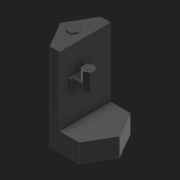
# Autodesk Inventor part: body
Saved by Autodesk Inventor 2017 (Build 210142000, 142)
## iProperties
Created: 2019-08-03
Part Number: body
Material: ABS Plastic
Document SubType Name: Modeling
Designer: Dell
Density: 1.06 g/cm^3
Appearance: Smooth - Black
Author: Dell
Autodesk Inventor part; units mm, degrees
ref_plane "YZ Plane" through (0, 0, 0) normal (1, 0, 0) x (0, 1, 0)
ref_plane "XZ Plane" through (0, 0, 0) normal (0, 1, 0) x (-1, 0, 0)
ref_plane "XY Plane" through (0, 0, 0) normal (0, 0, 1) x (1, 0, 0)
sketch "Sketch1" plane through (0, 0, 0) normal (0, 0, 1) x (1, 0, 0)
  line L0 (303.011, 0) -> (151.5055, -262.4152)
  line L1 (151.5055, -262.4152) -> (-151.5055, -262.4152)
  line L2 (-151.5055, -262.4152) -> (-303.011, 0)
  line L3 (-303.011, 0) -> (-151.5055, 262.4152)
  line L4 (-151.5055, 262.4152) -> (151.5055, 262.4152)
  line L5 (151.5055, 262.4152) -> (303.011, 0)
  point P0 (0, 0)
  point P1 (0, 0)
  dimension "d0" = 606.022
  constraints: 12 end point, 1 coincident, 1 horizontal alignment, 13 other
  measures "d0" distance of L2.end L0.start
extrude "Extrusion1" add sketch "Sketch1" along normal blind 190.5
sketch "Sketch2" plane through (0, 0, 190.5) normal (0, 0, 1) x (1, 0, 0)
  line L0 (151.5055, -262.4152) -> (303.011, 0) projected
  line L1 (303.011, 0) -> (151.5055, 262.4152) projected
  line L2 (151.5055, 262.4152) -> (-151.5055, 262.4152) construction
  line L3 (-151.5055, 262.4152) -> (-303.011, 0) projected
  line L4 (-303.011, 0) -> (-151.5055, -262.4152) projected
  line L5 (-151.5055, -262.4152) -> (151.5055, -262.4152) construction
  line L6 (151.5055, 262.4152) -> (-151.5055, 262.4152) projected
  line L7 (-50.7278, 262.4152) -> (-50.7278, -262.4152)
  line L8 (-151.5055, -262.4152) -> (151.5055, -262.4152) projected
  line L9 (-50.7278, 262.4152) -> (-151.5055, 262.4152)
  line L10 (-50.7278, -262.4152) -> (-151.5055, -262.4152)
  point P0 (0, 0)
  dimension "d3" = 353.7388
  constraints: 6 end point, 2 collinear, 2 point on line, 1 perpendicular
  measures "d3" distance from line of L0.end L7
extrude "Extrusion2" add sketch "Sketch2" along normal blind 704.85 contours L8 L4 L3 L6 L7
sketch "Sketch3" plane through (-50.7278, -262.4152, 190.5) normal (1, 0, 0) x (0, 0, -1)
  line L0 (-428.7, 86.64) -> (-358.7, 86.64)
  line L1 (-358.7, 86.64) -> (-358.7, 251.64)
  line L2 (-358.7, 251.64) -> (-428.7, 251.64)
  line L3 (-428.7, 251.64) -> (-428.7, 86.64)
  line L4 (0, 0) -> (-704.85, 0) projected
  line L5 (0, 0) -> (0, 262.4152) projected
  point P0 (190.5, 262.4152)
  dimension "d6" = 86.64
  dimension "d7" = 358.7
  dimension "d8" = 70
  dimension "d9" = 165
  constraints: 8 end point, 2 parallel, 1 horizontal, 1 perpendicular
  measures "d6" distance between parallel lines of L0 L4
  measures "d7" distance between parallel lines of L5 L1
  measures "d8" distance of L0.start L0.end
  measures "d9" distance of L2.end L0.start
extrude "Extrusion3" add sketch "Sketch3" along normal blind 30
sketch "Sketch4" plane through (-20.7278, -262.4152, 190.5) normal (1, 0, 0) x (0, 0, -1)
  line L0 (-428.7, 86.64) -> (-428.7, 251.64) projected
  line L1 (-358.7, 251.64) -> (-358.7, 86.64) projected
  line L2 (-428.7, 111.64) -> (-358.7, 111.64)
  line L3 (-358.7, 111.64) -> (-358.7, 226.64)
  line L4 (-358.7, 226.64) -> (-428.7, 226.64)
  line L5 (-428.7, 226.64) -> (-428.7, 111.64)
  point P0 (190.5, 262.4152)
  point P1 (-428.7, 169.14)
  dimension "d12" = 115
  constraints: 8 end point, 2 midpoint, 2 parallel, 2 point on line, 1 horizontal, 1 perpendicular
  measures "d12" distance between parallel lines of L4 L2
extrude "Extrusion4" add sketch "Sketch4" along normal blind 98.2
sketch "Sketch5" plane through (-50.7278, -175.7752, 619.2) normal (0, 0, 1) x (1, 0, 0)
  line L0 (128.2, 25) -> (128.2, 140) projected
  line L1 (128.2, 140) -> (177.9965, 111.25)
  line L2 (177.9965, 111.25) -> (177.9965, 53.75)
  line L3 (177.9965, 53.75) -> (128.2, 25)
  line L4 (128.2, 25) -> (78.4035, 53.75)
  line L5 (78.4035, 53.75) -> (78.4035, 111.25)
  line L6 (78.4035, 111.25) -> (128.2, 140)
  point P0 (50.7278, 175.7752)
  point P1 (128.2, 82.5)
  constraints: 12 end point, 1 midpoint, 13 other
extrude "Extrusion5" add sketch "Sketch5" along normal blind 110 and the other way blind 70
sketch "Sketch6" plane through (0, 0, 895.35) normal (0, 0, 1) x (1, 0, 0)
  line L0 (-115.8774, 0) -> (-144.6274, -49.7965)
  line L1 (-144.6274, -49.7965) -> (-202.1274, -49.7965)
  line L2 (-202.1274, -49.7965) -> (-230.8774, 0)
  line L3 (-230.8774, 0) -> (-202.1274, 49.7965)
  line L4 (-202.1274, 49.7965) -> (-144.6274, 49.7965)
  line L5 (-144.6274, 49.7965) -> (-115.8774, 0)
  line L6 (-50.7278, -262.4152) -> (-50.7278, 262.4152) projected
  point P0 (0, 0)
  point P1 (-173.3774, 0)
  point P2 (-50.7278, 0)
  dimension "d19" = 115
  dimension "d20" = 122.6496
  constraints: 12 end point, 2 horizontal alignment, 1 midpoint, 13 other
  measures "d19" distance of L0.start L2.end
  measures "d20" distance from line of L6 point (-173.377, 0)
extrude "Extrusion6" add sketch "Sketch6" along normal blind 11.725
sketch "Sketch7" plane through (-50.7278, -175.7752, 729.2) normal (0, 0, 1) x (1, 0, 0)
  line L0 (177.9965, 111.25) -> (128.2, 140) projected
  line L1 (128.2, 140) -> (78.4035, 111.25) projected
  line L2 (78.4035, 111.25) -> (78.4035, 53.75) projected
  line L3 (78.4035, 53.75) -> (128.2, 25) projected
  line L4 (128.2, 25) -> (177.9965, 53.75) projected
  line L5 (177.9965, 53.75) -> (177.9965, 111.25) projected
  circle A0 centre (128.2, 82.5) radius 25
  point P0 (50.7278, 175.7752)
  point P1 (177.9965, 82.5)
  dimension "d23" = 50
  constraints: 1 centre point, 1 horizontal alignment, 1 midpoint, 1 vertical alignment
  measures "d23" diameter of A0
extrude "Extrusion7" add sketch "Sketch7" along normal blind 5 contours A0
sketch "Sketch8" plane through (-151.5055, -262.4152, 0) normal (0, -1, 0) x (1, 0, 0)
  line L0 (303.011, 0) -> (0, 0) projected
  line L1 (303.011, 0) -> (303.011, 190.5) projected
  line L2 (100.7777, 190.5) -> (303.011, 190.5) projected
  line L3 (100.7777, 190.5) -> (100.7777, 895.35) projected
  line L4 (0, 895.35) -> (100.7777, 895.35) projected
  line L5 (0, 0) -> (0, 895.35) projected
  circle A0 centre (251.021, 50.8) radius 4
  point P0 (151.5055, 0)
  dimension "d26" = 8
  dimension "d27" = 50.8
  dimension "d28" = 51.99
  constraints: 1 centre point
  measures "d26" diameter of A0
  measures "d27" distance from line of L0 A0.centre
  measures "d28" distance from line of L1 A0.centre
extrude "Extrusion8" cut sketch "Sketch8" against normal through all contours A0
sketch "Sketch9" plane through (0, 0, 0) normal (0, 0, -1) x (-1, 0, 0)
  circle A0 centre (246.7476, 0) radius 5
  point P0 (0, 0)
  point P1 (303.011, 0)
  dimension "d31" = 10
  dimension "d32" = 56.2634
  constraints: 1 centre point, 1 horizontal alignment
  measures "d31" diameter of A0
  measures "d32" distance of point (303.011, 0) A0.centre
extrude "Extrusion9" add sketch "Sketch9" along normal blind 5
body "Solid1"
